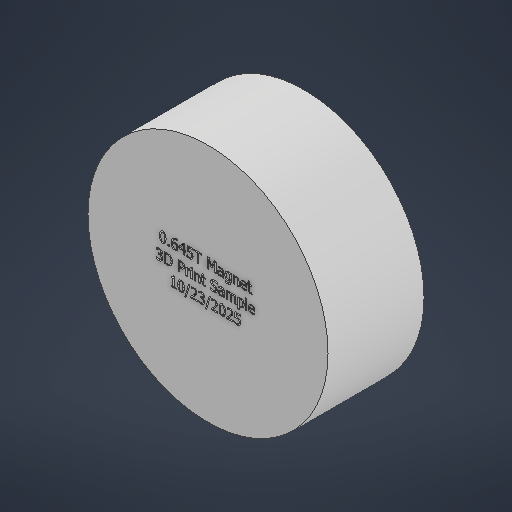
# Autodesk Inventor part: Sample_Magnet
Saved by Autodesk Inventor 2026.1 (Build 301233000, 233)
## iProperties
Created: 2025-10-23
Part Number: Sample_Magnet
Material: Generic
Document SubType Name: Modeling
Designer: usman
Density: 1 g/cm^3
Appearance: Default
Author: usman
Autodesk Inventor part; units mm, degrees
ref_plane "YZ Plane" through (0, 0, 0) normal (1, 0, 0) x (0, 1, 0)
ref_plane "XZ Plane" through (0, 0, 0) normal (0, 1, 0) x (-1, 0, 0)
ref_plane "XY Plane" through (0, 0, 0) normal (0, 0, 1) x (1, 0, 0)
sketch "Sketch1" plane through (0, 0, 0) normal (0, 0, 1) x (1, 0, 0)
  circle A0 centre (0, 0) radius 37.5
  dimension "d0" = 75
  constraints: 1 centre point, 1 coincident
  measures "d0" diameter of A0
extrude "Extrusion1" add sketch "Sketch1" along normal blind 30
sketch "Sketch2" plane through (0, 0, 30) normal (0, 0, 1) x (1, 0, 0)
  line L0 (-22.0603, 24.5034) -> (20.4794, 24.5034) construction
  line L1 (20.4794, 24.5034) -> (20.4794, -24.5034) construction
  line L2 (20.4794, -24.5034) -> (-22.0603, -24.5034) construction
  line L3 (-22.0603, -24.5034) -> (-22.0603, 24.5034) construction
  spline S0 degree 2 poles (-13.0981, 5.5402) (-13.0981, 4.686) (-13.5946, 3.8858) (-14.1118, 3.8858) knots 0 0 0 1 2 2 2
  spline S1 degree 2 poles (-14.1118, 3.8858) (-14.6367, 3.8858) (-15.1281, 4.7014) (-15.1281, 5.5376) knots 0 0 0 1 2 2 2
  spline S2 degree 2 poles (-15.1281, 5.5376) (-15.1281, 6.397) (-14.6315, 7.192) (-14.1118, 7.192) knots 0 0 0 1 2 2 2
  spline S3 degree 2 poles (-14.1118, 7.192) (-13.5895, 7.192) (-13.0981, 6.3686) (-13.0981, 5.5402) knots 0 0 0 1 2 2 2
  spline S4 degree 2 poles (-13.6435, 4.5727) (-13.5818, 4.7297) (-13.5303, 5.2134) (-13.5303, 5.5402) knots 0 0 0 1 2 2 2
  spline S5 degree 2 poles (-13.5303, 5.5402) (-13.5303, 5.8669) (-13.5818, 6.3481) (-13.6461, 6.5102) knots 0 0 0 1 2 2 2
  spline S6 degree 2 poles (-13.6461, 6.5102) (-13.7104, 6.6723) (-13.9343, 6.8395) (-14.1118, 6.8395) knots 0 0 0 1 2 2 2
  spline S7 degree 2 poles (-14.1118, 6.8395) (-14.2893, 6.8395) (-14.5183, 6.6723) (-14.5852, 6.505) knots 0 0 0 1 2 2 2
  spline S8 degree 2 poles (-14.5852, 6.505) (-14.6495, 6.3429) (-14.6959, 5.8489) (-14.6959, 5.5376) knots 0 0 0 1 2 2 2
  spline S9 degree 2 poles (-14.6959, 5.5376) (-14.6959, 5.2031) (-14.6547, 4.7554) (-14.5878, 4.5805) knots 0 0 0 1 2 2 2
  spline S10 degree 2 poles (-14.5878, 4.5805) (-14.526, 4.4158) (-14.297, 4.2383) (-14.1118, 4.2383) knots 0 0 0 1 2 2 2
  spline S11 degree 2 poles (-14.1118, 4.2383) (-13.9368, 4.2383) (-13.7078, 4.4055) (-13.6435, 4.5727) knots 0 0 0 1 2 2 2
  line L4 (-12.0097, 3.9527) -> (-12.5192, 3.9527)
  line L5 (-12.5192, 3.9527) -> (-12.5192, 4.5599)
  line L6 (-12.5192, 4.5599) -> (-12.0097, 4.5599)
  line L7 (-12.0097, 4.5599) -> (-12.0097, 3.9527)
  spline S12 degree 2 poles (-9.3622, 4.9818) (-9.3622, 4.7374) (-9.5243, 4.3232) (-9.6606, 4.1842) knots 0 0 0 1 2 2 2
  spline S13 degree 2 poles (-9.6606, 4.1842) (-9.8021, 4.0376) (-10.1572, 3.8858) (-10.3708, 3.8858) knots 0 0 0 1 2 2 2
  spline S14 degree 2 poles (-10.3708, 3.8858) (-10.5843, 3.8858) (-10.9368, 4.0299) (-11.0706, 4.1739) knots 0 0 0 1 2 2 2
  spline S15 degree 2 poles (-11.0706, 4.1739) (-11.2353, 4.3463) (-11.4205, 4.9252) (-11.4205, 5.3472) knots 0 0 0 1 2 2 2
  spline S16 degree 2 poles (-11.4205, 5.3472) (-11.4205, 5.7614) (-11.2507, 6.4278) (-11.0732, 6.6748) knots 0 0 0 1 2 2 2
  spline S17 degree 2 poles (-11.0732, 6.6748) (-10.9008, 6.9167) (-10.3553, 7.1868) (-9.9977, 7.1868) knots 0 0 0 1 2 2 2
  spline S18 degree 2 poles (-9.9977, 7.1868) (-9.8922, 7.1868) (-9.7069, 7.1663) (-9.6375, 7.1431) knots 0 0 0 1 2 2 2
  line L8 (-9.6375, 7.1431) -> (-9.6375, 6.734)
  line L9 (-9.6375, 6.734) -> (-9.6555, 6.734)
  spline S19 degree 2 poles (-9.6555, 6.734) (-9.7147, 6.7649) (-9.9308, 6.8189) (-10.0543, 6.8189) knots 0 0 0 1 2 2 2
  spline S20 degree 2 poles (-10.0543, 6.8189) (-10.4505, 6.8189) (-10.9368, 6.2837) (-10.9831, 5.7589) knots 0 0 0 1 2 2 2
  spline S21 degree 2 poles (-10.9831, 5.7589) (-10.8313, 5.8644) (-10.5123, 5.9801) (-10.3219, 5.9801) knots 0 0 0 1 2 2 2
  spline S22 degree 2 poles (-10.3219, 5.9801) (-10.1366, 5.9801) (-9.8587, 5.9055) (-9.7069, 5.7923) knots 0 0 0 1 2 2 2
  spline S23 degree 2 poles (-9.7069, 5.7923) (-9.532, 5.6611) (-9.3622, 5.2546) (-9.3622, 4.9818) knots 0 0 0 1 2 2 2
  spline S24 degree 2 poles (-9.7944, 4.9638) (-9.7944, 5.1594) (-9.8973, 5.4244) (-10.0105, 5.517) knots 0 0 0 1 2 2 2
  spline S25 degree 2 poles (-10.0105, 5.517) (-10.0954, 5.5839) (-10.3064, 5.6276) (-10.4171, 5.6276) knots 0 0 0 1 2 2 2
  spline S26 degree 2 poles (-10.4171, 5.6276) (-10.5663, 5.6276) (-10.8467, 5.5376) (-10.9831, 5.4527) knots 0 0 0 1 2 2 2
  spline S27 degree 2 poles (-10.9831, 5.4527) (-10.9857, 5.4064) (-10.9908, 5.3189) (-10.9908, 5.252) knots 0 0 0 1 2 2 2
  spline S28 degree 2 poles (-10.9908, 5.252) (-10.9908, 4.9227) (-10.8622, 4.5187) (-10.7644, 4.4132) knots 0 0 0 1 2 2 2
  spline S29 degree 2 poles (-10.7644, 4.4132) (-10.6744, 4.3129) (-10.4788, 4.2331) (-10.3682, 4.2331) knots 0 0 0 1 2 2 2
  spline S30 degree 2 poles (-10.3682, 4.2331) (-10.1109, 4.2331) (-9.7944, 4.5985) (-9.7944, 4.9638) knots 0 0 0 1 2 2 2
  line L10 (-6.9436, 5.0436) -> (-7.3218, 5.0436)
  line L11 (-7.3218, 5.0436) -> (-7.3218, 3.9527)
  line L12 (-7.3218, 3.9527) -> (-7.7309, 3.9527)
  line L13 (-7.7309, 3.9527) -> (-7.7309, 5.0436)
  line L14 (-7.7309, 5.0436) -> (-9.1332, 5.0436)
  line L15 (-9.1332, 5.0436) -> (-9.1332, 5.4913)
  line L16 (-9.1332, 5.4913) -> (-7.7129, 7.1277)
  line L17 (-7.7129, 7.1277) -> (-7.3218, 7.1277)
  line L18 (-7.3218, 7.1277) -> (-7.3218, 5.3858)
  line L19 (-7.3218, 5.3858) -> (-6.9436, 5.3858)
  line L20 (-6.9436, 5.3858) -> (-6.9436, 5.0436)
  line L21 (-7.7309, 5.3858) -> (-7.7309, 6.6259)
  line L22 (-7.7309, 6.6259) -> (-8.7987, 5.3858)
  line L23 (-8.7987, 5.3858) -> (-7.7309, 5.3858)
  spline S31 degree 2 poles (-4.6794, 4.9613) (-4.6794, 4.7323) (-4.8261, 4.3412) (-4.9599, 4.1971) knots 0 0 0 1 2 2 2
  spline S32 degree 2 poles (-4.9599, 4.1971) (-5.0937, 4.053) (-5.4925, 3.8858) (-5.7395, 3.8858) knots 0 0 0 1 2 2 2
  spline S33 degree 2 poles (-5.7395, 3.8858) (-5.9659, 3.8858) (-6.4084, 3.9861) (-6.5705, 4.0659) knots 0 0 0 1 2 2 2
  line L24 (-6.5705, 4.0659) -> (-6.5705, 4.5161)
  line L25 (-6.5705, 4.5161) -> (-6.5397, 4.5161)
  spline S34 degree 2 poles (-6.5397, 4.5161) (-6.4908, 4.4801) (-6.3081, 4.3875) (-6.1975, 4.3463) knots 0 0 0 1 2 2 2
  spline S35 degree 2 poles (-6.1975, 4.3463) (-6.0714, 4.3026) (-5.863, 4.2537) (-5.7318, 4.2537) knots 0 0 0 1 2 2 2
  spline S36 degree 2 poles (-5.7318, 4.2537) (-5.6031, 4.2537) (-5.3612, 4.3463) (-5.2738, 4.4467) knots 0 0 0 1 2 2 2
  spline S37 degree 2 poles (-5.2738, 4.4467) (-5.194, 4.5419) (-5.1117, 4.794) (-5.1117, 4.9638) knots 0 0 0 1 2 2 2
  spline S38 degree 2 poles (-5.1117, 4.9638) (-5.1117, 5.1336) (-5.2043, 5.3498) (-5.2918, 5.4218) knots 0 0 0 1 2 2 2
  spline S39 degree 2 poles (-5.2918, 5.4218) (-5.3818, 5.5016) (-5.6494, 5.5685) (-5.8115, 5.5685) knots 0 0 0 1 2 2 2
  spline S40 degree 2 poles (-5.8115, 5.5685) (-5.9865, 5.5685) (-6.3338, 5.5144) (-6.4393, 5.4913) knots 0 0 0 1 2 2 2
  line L26 (-6.4393, 5.4913) -> (-6.4393, 7.1277)
  line L27 (-6.4393, 7.1277) -> (-4.6974, 7.1277)
  line L28 (-4.6974, 7.1277) -> (-4.6974, 6.7546)
  line L29 (-4.6974, 6.7546) -> (-6.0302, 6.7546)
  line L30 (-6.0302, 6.7546) -> (-6.0302, 5.9081)
  spline S41 degree 2 poles (-6.0302, 5.9081) (-5.953, 5.9184) (-5.8038, 5.9261) (-5.742, 5.9261) knots 0 0 0 1 2 2 2
  spline S42 degree 2 poles (-5.742, 5.9261) (-5.4976, 5.9261) (-5.1606, 5.8463) (-5.0062, 5.728) knots 0 0 0 1 2 2 2
  spline S43 degree 2 poles (-5.0062, 5.728) (-4.8492, 5.6096) (-4.6794, 5.2494) (-4.6794, 4.9613) knots 0 0 0 1 2 2 2
  line L31 (-3.3904, 3.9527) -> (-3.3904, 6.752)
  line L32 (-3.3904, 6.752) -> (-4.4556, 6.752)
  line L33 (-4.4556, 6.752) -> (-4.4556, 7.1277)
  line L34 (-4.4556, 7.1277) -> (-1.9032, 7.1277)
  line L35 (-1.9032, 7.1277) -> (-1.9032, 6.752)
  line L36 (-1.9032, 6.752) -> (-2.9684, 6.752)
  line L37 (-2.9684, 6.752) -> (-2.9684, 3.9527)
  line L38 (-2.9684, 3.9527) -> (-3.3904, 3.9527)
  line L39 (2.5042, 3.9527) -> (2.0822, 3.9527)
  line L40 (2.0822, 3.9527) -> (2.0822, 6.6877)
  line L41 (2.0822, 6.6877) -> (1.2538, 4.8275)
  line L42 (1.2538, 4.8275) -> (0.9965, 4.8275)
  line L43 (0.9965, 4.8275) -> (0.1757, 6.6877)
  line L44 (0.1757, 6.6877) -> (0.1757, 3.9527)
  line L45 (0.1757, 3.9527) -> (-0.218, 3.9527)
  line L46 (-0.218, 3.9527) -> (-0.218, 7.1277)
  line L47 (-0.218, 7.1277) -> (0.3584, 7.1277)
  line L48 (0.3584, 7.1277) -> (1.1508, 5.3601)
  line L49 (1.1508, 5.3601) -> (1.9176, 7.1277)
  line L50 (1.9176, 7.1277) -> (2.5042, 7.1277)
  line L51 (2.5042, 7.1277) -> (2.5042, 3.9527)
  spline S44 degree 2 poles (4.4442, 4.2048) (4.3953, 4.1688) (4.2306, 4.0401) (4.1535, 4.0016) knots 0 0 0 1 2 2 2
  spline S45 degree 2 poles (4.1535, 4.0016) (4.048, 3.9449) (3.8499, 3.8858) (3.6697, 3.8858) knots 0 0 0 1 2 2 2
  spline S46 degree 2 poles (3.6697, 3.8858) (3.5231, 3.8858) (3.2581, 3.9964) (3.1577, 4.0967) knots 0 0 0 1 2 2 2
  spline S47 degree 2 poles (3.1577, 4.0967) (3.0625, 4.1945) (2.9468, 4.4827) (2.9468, 4.6422) knots 0 0 0 1 2 2 2
  spline S48 degree 2 poles (2.9468, 4.6422) (2.9468, 4.8892) (3.1552, 5.2391) (3.3816, 5.3395) knots 0 0 0 1 2 2 2
  spline S49 degree 2 poles (3.3816, 5.3395) (3.5823, 5.4321) (4.1277, 5.5016) (4.4442, 5.5196) knots 0 0 0 1 2 2 2
  line L52 (4.4442, 5.5196) -> (4.4442, 5.5968)
  spline S50 degree 2 poles (4.4442, 5.5968) (4.4442, 5.7357) (4.3593, 5.9081) (4.2821, 5.957) knots 0 0 0 1 2 2 2
  spline S51 degree 2 poles (4.2821, 5.957) (4.2049, 6.0059) (3.9836, 6.0367) (3.8653, 6.0367) knots 0 0 0 1 2 2 2
  spline S52 degree 2 poles (3.8653, 6.0367) (3.7264, 6.0367) (3.3507, 5.9544) (3.1629, 5.8746) knots 0 0 0 1 2 2 2
  line L53 (3.1629, 5.8746) -> (3.1397, 5.8746)
  line L54 (3.1397, 5.8746) -> (3.1397, 6.2837)
  spline S53 degree 2 poles (3.1397, 6.2837) (3.2504, 6.3146) (3.6646, 6.3918) (3.8679, 6.3918) knots 0 0 0 1 2 2 2
  spline S54 degree 2 poles (3.8679, 6.3918) (4.1149, 6.3918) (4.4519, 6.3146) (4.5857, 6.2143) knots 0 0 0 1 2 2 2
  spline S55 degree 2 poles (4.5857, 6.2143) (4.7169, 6.1165) (4.8456, 5.8052) (4.8456, 5.5813) knots 0 0 0 1 2 2 2
  line L55 (4.8456, 5.5813) -> (4.8456, 3.9527)
  line L56 (4.8456, 3.9527) -> (4.4442, 3.9527)
  line L57 (4.4442, 3.9527) -> (4.4442, 4.2048)
  line L58 (4.4442, 4.5393) -> (4.4442, 5.2005)
  spline S56 degree 2 poles (4.4442, 5.2005) (4.3001, 5.1877) (3.8653, 5.1439) (3.7289, 5.1028) knots 0 0 0 1 2 2 2
  spline S57 degree 2 poles (3.7289, 5.1028) (3.5694, 5.0539) (3.361, 4.8506) (3.361, 4.6705) knots 0 0 0 1 2 2 2
  spline S58 degree 2 poles (3.361, 4.6705) (3.361, 4.4647) (3.5926, 4.2563) (3.8138, 4.2563) knots 0 0 0 1 2 2 2
  spline S59 degree 2 poles (3.8138, 4.2563) (4.0017, 4.2563) (4.3104, 4.4184) (4.4442, 4.5393) knots 0 0 0 1 2 2 2
  spline S60 degree 2 poles (5.494, 3.5719) (5.5351, 3.5539) (5.6921, 3.4973) (5.7924, 3.4741) knots 0 0 0 1 2 2 2
  spline S61 degree 2 poles (5.7924, 3.4741) (5.9031, 3.4458) (6.0909, 3.4123) (6.2015, 3.4123) knots 0 0 0 1 2 2 2
  spline S62 degree 2 poles (6.2015, 3.4123) (6.3868, 3.4123) (6.6441, 3.5101) (6.7161, 3.5976) knots 0 0 0 1 2 2 2
  spline S63 degree 2 poles (6.7161, 3.5976) (6.7856, 3.6851) (6.8396, 3.9141) (6.8396, 4.0607) knots 0 0 0 1 2 2 2
  line L59 (6.8396, 4.0607) -> (6.8396, 4.2691)
  spline S64 degree 2 poles (6.8396, 4.2691) (6.6775, 4.1276) (6.3662, 3.9938) (6.132, 3.9938) knots 0 0 0 1 2 2 2
  spline S65 degree 2 poles (6.132, 3.9938) (5.7255, 3.9938) (5.2444, 4.5985) (5.2444, 5.1671) knots 0 0 0 1 2 2 2
  spline S66 degree 2 poles (5.2444, 5.1671) (5.2444, 5.463) (5.4116, 5.921) (5.5506, 6.0831) knots 0 0 0 1 2 2 2
  spline S67 degree 2 poles (5.5506, 6.0831) (5.6844, 6.2349) (6.0523, 6.4021) (6.2478, 6.4021) knots 0 0 0 1 2 2 2
  spline S68 degree 2 poles (6.2478, 6.4021) (6.4331, 6.4021) (6.7032, 6.3146) (6.8396, 6.2349) knots 0 0 0 1 2 2 2
  line L60 (6.8396, 6.2349) -> (6.8628, 6.3352)
  line L61 (6.8628, 6.3352) -> (7.241, 6.3352)
  line L62 (7.241, 6.3352) -> (7.241, 4.2254)
  spline S69 degree 2 poles (7.241, 4.2254) (7.241, 3.6182) (6.7135, 3.0521) (6.1706, 3.0521) knots 0 0 0 1 2 2 2
  spline S70 degree 2 poles (6.1706, 3.0521) (5.9957, 3.0521) (5.6303, 3.1087) (5.4734, 3.1551) knots 0 0 0 1 2 2 2
  line L63 (5.4734, 3.1551) -> (5.4734, 3.5719)
  line L64 (5.4734, 3.5719) -> (5.494, 3.5719)
  line L65 (6.8396, 4.5985) -> (6.8396, 5.9081)
  spline S71 degree 2 poles (6.8396, 5.9081) (6.6904, 5.9801) (6.4382, 6.0419) (6.3122, 6.0419) knots 0 0 0 1 2 2 2
  spline S72 degree 2 poles (6.3122, 6.0419) (6.0085, 6.0419) (5.6586, 5.5942) (5.6586, 5.1748) knots 0 0 0 1 2 2 2
  spline S73 degree 2 poles (5.6586, 5.1748) (5.6586, 4.7786) (5.9236, 4.3643) (6.2221, 4.3643) knots 0 0 0 1 2 2 2
  spline S74 degree 2 poles (6.2221, 4.3643) (6.379, 4.3643) (6.7084, 4.4878) (6.8396, 4.5985) knots 0 0 0 1 2 2 2
  line L66 (9.693, 3.9527) -> (9.2916, 3.9527)
  line L67 (9.2916, 3.9527) -> (9.2916, 5.3112)
  spline S75 degree 2 poles (9.2916, 5.3112) (9.2916, 5.4758) (9.2607, 5.7589) (9.2144, 5.8438) knots 0 0 0 1 2 2 2
  spline S76 degree 2 poles (9.2144, 5.8438) (9.1655, 5.9338) (8.9906, 6.0213) (8.8413, 6.0213) knots 0 0 0 1 2 2 2
  spline S77 degree 2 poles (8.8413, 6.0213) (8.6921, 6.0213) (8.3756, 5.8618) (8.2238, 5.7331) knots 0 0 0 1 2 2 2
  line L68 (8.2238, 5.7331) -> (8.2238, 3.9527)
  line L69 (8.2238, 3.9527) -> (7.8225, 3.9527)
  line L70 (7.8225, 3.9527) -> (7.8225, 6.3352)
  line L71 (7.8225, 6.3352) -> (8.2238, 6.3352)
  line L72 (8.2238, 6.3352) -> (8.2238, 6.0702)
  spline S78 degree 2 poles (8.2238, 6.0702) (8.4039, 6.2323) (8.7513, 6.4021) (8.9468, 6.4021) knots 0 0 0 1 2 2 2
  spline S79 degree 2 poles (8.9468, 6.4021) (9.2968, 6.4021) (9.693, 5.939) (9.693, 5.499) knots 0 0 0 1 2 2 2
  line L73 (9.693, 5.499) -> (9.693, 3.9527)
  spline S80 degree 2 poles (11.2908, 3.8986) (10.7196, 3.8986) (10.0918, 4.5393) (10.0918, 5.1311) knots 0 0 0 1 2 2 2
  spline S81 degree 2 poles (10.0918, 5.1311) (10.0918, 5.7126) (10.7016, 6.4021) (11.193, 6.4021) knots 0 0 0 1 2 2 2
  spline S82 degree 2 poles (11.193, 6.4021) (11.4143, 6.4021) (11.7565, 6.2735) (11.8826, 6.1371) knots 0 0 0 1 2 2 2
  spline S83 degree 2 poles (11.8826, 6.1371) (12.0112, 6.0007) (12.1476, 5.6071) (12.1476, 5.3215) knots 0 0 0 1 2 2 2
  line L74 (12.1476, 5.3215) -> (12.1476, 5.1028)
  line L75 (12.1476, 5.1028) -> (10.4983, 5.1028)
  spline S84 degree 2 poles (10.4983, 5.1028) (10.4983, 4.6885) (10.9151, 4.2486) (11.2856, 4.2486) knots 0 0 0 1 2 2 2
  spline S85 degree 2 poles (11.2856, 4.2486) (11.4169, 4.2486) (11.6716, 4.3077) (11.7745, 4.354) knots 0 0 0 1 2 2 2
  spline S86 degree 2 poles (11.7745, 4.354) (11.8826, 4.4055) (12.0318, 4.4956) (12.0807, 4.5367) knots 0 0 0 1 2 2 2
  line L76 (12.0807, 4.5367) -> (12.1038, 4.5367)
  line L77 (12.1038, 4.5367) -> (12.1038, 4.0993)
  spline S87 degree 2 poles (12.1038, 4.0993) (12.0344, 4.071) (11.8234, 3.9887) (11.741, 3.9655) knots 0 0 0 1 2 2 2
  spline S88 degree 2 poles (11.741, 3.9655) (11.6253, 3.9321) (11.4349, 3.8986) (11.2908, 3.8986) knots 0 0 0 1 2 2 2
  spline S89 degree 2 poles (11.7565, 5.4089) (11.7513, 5.571) (11.6844, 5.8078) (11.6201, 5.8875) knots 0 0 0 1 2 2 2
  spline S90 degree 2 poles (11.6201, 5.8875) (11.5506, 5.9776) (11.3319, 6.0728) (11.1698, 6.0728) knots 0 0 0 1 2 2 2
  spline S91 degree 2 poles (11.1698, 6.0728) (11.0103, 6.0728) (10.7865, 5.9776) (10.6939, 5.8849) knots 0 0 0 1 2 2 2
  spline S92 degree 2 poles (10.6939, 5.8849) (10.6038, 5.7897) (10.5112, 5.5607) (10.4983, 5.4089) knots 0 0 0 1 2 2 2
  line L78 (10.4983, 5.4089) -> (11.7565, 5.4089)
  spline S93 degree 2 poles (13.2745, 3.9064) (12.9477, 3.9064) (12.5798, 4.2794) (12.5798, 4.6834) knots 0 0 0 1 2 2 2
  line L79 (12.5798, 4.6834) -> (12.5798, 6.0033)
  line L80 (12.5798, 6.0033) -> (12.3097, 6.0033)
  line L81 (12.3097, 6.0033) -> (12.3097, 6.3352)
  line L82 (12.3097, 6.3352) -> (12.5798, 6.3352)
  line L83 (12.5798, 6.3352) -> (12.5798, 7.0196)
  line L84 (12.5798, 7.0196) -> (12.9812, 7.0196)
  line L85 (12.9812, 7.0196) -> (12.9812, 6.3352)
  line L86 (12.9812, 6.3352) -> (13.7196, 6.3352)
  line L87 (13.7196, 6.3352) -> (13.7196, 6.0033)
  line L88 (13.7196, 6.0033) -> (12.9812, 6.0033)
  line L89 (12.9812, 6.0033) -> (12.9812, 4.8686)
  spline S94 degree 2 poles (12.9812, 4.8686) (12.9812, 4.6885) (12.9941, 4.4904) (13.0378, 4.4055) knots 0 0 0 1 2 2 2
  spline S95 degree 2 poles (13.0378, 4.4055) (13.0738, 4.3309) (13.2359, 4.2563) (13.3749, 4.2563) knots 0 0 0 1 2 2 2
  spline S96 degree 2 poles (13.3749, 4.2563) (13.4726, 4.2563) (13.6553, 4.3154) (13.6965, 4.3335) knots 0 0 0 1 2 2 2
  line L90 (13.6965, 4.3335) -> (13.7196, 4.3335)
  line L91 (13.7196, 4.3335) -> (13.7196, 3.9732)
  spline S97 degree 2 poles (13.7196, 3.9732) (13.6064, 3.9424) (13.3749, 3.9064) (13.2745, 3.9064) knots 0 0 0 1 2 2 2
  spline S98 degree 2 poles (-15.2259, 1.5991) (-15.3417, 1.5991) (-15.5706, 1.5425) (-15.6813, 1.4987) knots 0 0 0 1 2 2 2
  spline S99 degree 2 poles (-15.6813, 1.4987) (-15.7842, 1.455) (-15.936, 1.3624) (-15.9952, 1.3212) knots 0 0 0 1 2 2 2
  line L92 (-15.9952, 1.3212) -> (-16.0209, 1.3212)
  line L93 (-16.0209, 1.3212) -> (-16.0209, 1.7715)
  spline S100 degree 2 poles (-16.0209, 1.7715) (-15.882, 1.8461) (-15.406, 1.967) (-15.1924, 1.967) knots 0 0 0 1 2 2 2
  spline S101 degree 2 poles (-15.1924, 1.967) (-14.9763, 1.967) (-14.6547, 1.8795) (-14.5235, 1.7869) knots 0 0 0 1 2 2 2
  spline S102 degree 2 poles (-14.5235, 1.7869) (-14.3845, 1.6866) (-14.2404, 1.3958) (-14.2404, 1.2003) knots 0 0 0 1 2 2 2
  spline S103 degree 2 poles (-14.2404, 1.2003) (-14.2404, 0.9378) (-14.5852, 0.5416) (-14.8271, 0.4901) knots 0 0 0 1 2 2 2
  line L94 (-14.8271, 0.4901) -> (-14.8271, 0.4593)
  spline S104 degree 2 poles (-14.8271, 0.4593) (-14.7267, 0.4387) (-14.4977, 0.3461) (-14.4, 0.2534) knots 0 0 0 1 2 2 2
  spline S105 degree 2 poles (-14.4, 0.2534) (-14.3022, 0.1634) (-14.1787, -0.1248) (-14.1787, -0.3332) knots 0 0 0 1 2 2 2
  spline S106 degree 2 poles (-14.1787, -0.3332) (-14.1787, -0.5467) (-14.3253, -0.9095) (-14.4591, -1.0485) knots 0 0 0 1 2 2 2
  spline S107 degree 2 poles (-14.4591, -1.0485) (-14.5981, -1.1926) (-14.9917, -1.3418) (-15.2413, -1.3418) knots 0 0 0 1 2 2 2
  spline S108 degree 2 poles (-15.2413, -1.3418) (-15.4806, -1.3418) (-15.9489, -1.226) (-16.1084, -1.1462) knots 0 0 0 1 2 2 2
  line L95 (-16.1084, -1.1462) -> (-16.1084, -0.696)
  line L96 (-16.1084, -0.696) -> (-16.0775, -0.696)
  spline S109 degree 2 poles (-16.0775, -0.696) (-15.9437, -0.7937) (-15.4909, -0.9739) (-15.267, -0.9739) knots 0 0 0 1 2 2 2
  spline S110 degree 2 poles (-15.267, -0.9739) (-15.1358, -0.9739) (-14.8734, -0.8915) (-14.7859, -0.7963) knots 0 0 0 1 2 2 2
  spline S111 degree 2 poles (-14.7859, -0.7963) (-14.701, -0.7011) (-14.6109, -0.4747) (-14.6109, -0.3023) knots 0 0 0 1 2 2 2
  spline S112 degree 2 poles (-14.6109, -0.3023) (-14.6109, -0.1299) (-14.7113, 0.0939) (-14.8013, 0.1582) knots 0 0 0 1 2 2 2
  spline S113 degree 2 poles (-14.8013, 0.1582) (-14.8914, 0.2226) (-15.1358, 0.2714) (-15.2799, 0.2714) knots 0 0 0 1 2 2 2
  line L97 (-15.2799, 0.2714) -> (-15.46, 0.2714)
  line L98 (-15.46, 0.2714) -> (-15.46, 0.6239)
  line L99 (-15.46, 0.6239) -> (-15.3185, 0.6239)
  spline S114 degree 2 poles (-15.3185, 0.6239) (-15.0329, 0.6239) (-14.6727, 0.8967) (-14.6727, 1.1565) knots 0 0 0 1 2 2 2
  spline S115 degree 2 poles (-14.6727, 1.1565) (-14.6727, 1.2775) (-14.7653, 1.4498) (-14.8399, 1.5013) knots 0 0 0 1 2 2 2
  spline S116 degree 2 poles (-14.8399, 1.5013) (-14.9197, 1.5553) (-15.1152, 1.5991) (-15.2259, 1.5991) knots 0 0 0 1 2 2 2
  spline S117 degree 2 poles (-11.1066, 0.31) (-11.1066, -0.1248) (-11.4591, -0.8246) (-11.755, -1.0202) knots 0 0 0 1 2 2 2
  spline S118 degree 2 poles (-11.755, -1.0202) (-11.9968, -1.172) (-12.4934, -1.2749) (-12.8794, -1.2749) knots 0 0 0 1 2 2 2
  line L100 (-12.8794, -1.2749) -> (-13.6101, -1.2749)
  line L101 (-13.6101, -1.2749) -> (-13.6101, 1.9001)
  line L102 (-13.6101, 1.9001) -> (-12.8871, 1.9001)
  spline S119 degree 2 poles (-12.8871, 1.9001) (-12.4394, 1.9001) (-11.9299, 1.7663) (-11.7498, 1.648) knots 0 0 0 1 2 2 2
  spline S120 degree 2 poles (-11.7498, 1.648) (-11.4437, 1.4447) (-11.1066, 0.7732) (-11.1066, 0.31) knots 0 0 0 1 2 2 2
  spline S121 degree 2 poles (-11.5466, 0.3152) (-11.5466, 0.6805) (-11.7884, 1.1977) (-12.0277, 1.3444) knots 0 0 0 1 2 2 2
  spline S122 degree 2 poles (-12.0277, 1.3444) (-12.1975, 1.4447) (-12.5809, 1.5348) (-12.8665, 1.5348) knots 0 0 0 1 2 2 2
  line L103 (-12.8665, 1.5348) -> (-13.1881, 1.5348)
  line L104 (-13.1881, 1.5348) -> (-13.1881, -0.9095)
  line L105 (-13.1881, -0.9095) -> (-12.8665, -0.9095)
  spline S123 degree 2 poles (-12.8665, -0.9095) (-12.586, -0.9095) (-12.1615, -0.8195) (-11.9891, -0.6986) knots 0 0 0 1 2 2 2
  spline S124 degree 2 poles (-11.9891, -0.6986) (-11.7679, -0.5493) (-11.5466, -0.0553) (-11.5466, 0.3152) knots 0 0 0 1 2 2 2
  spline S125 degree 2 poles (-7.2781, 0.943) (-7.2781, 0.7371) (-7.4247, 0.3666) (-7.556, 0.238) knots 0 0 0 1 2 2 2
  spline S126 degree 2 poles (-7.556, 0.238) (-7.7206, 0.0759) (-8.1657, -0.0913) (-8.5054, -0.0913) knots 0 0 0 1 2 2 2
  line L106 (-8.5054, -0.0913) -> (-8.863, -0.0913)
  line L107 (-8.863, -0.0913) -> (-8.863, -1.2749)
  line L108 (-8.863, -1.2749) -> (-9.285, -1.2749)
  line L109 (-9.285, -1.2749) -> (-9.285, 1.9001)
  line L110 (-9.285, 1.9001) -> (-8.4874, 1.9001)
  spline S127 degree 2 poles (-8.4874, 1.9001) (-8.2043, 1.9001) (-7.8081, 1.8075) (-7.6563, 1.702) knots 0 0 0 1 2 2 2
  spline S128 degree 2 poles (-7.6563, 1.702) (-7.4788, 1.5811) (-7.2781, 1.208) (-7.2781, 0.943) knots 0 0 0 1 2 2 2
  spline S129 degree 2 poles (-7.7181, 0.9301) (-7.7181, 1.0948) (-7.8313, 1.3366) (-7.947, 1.4138) knots 0 0 0 1 2 2 2
  spline S130 degree 2 poles (-7.947, 1.4138) (-8.0474, 1.4807) (-8.315, 1.5348) (-8.5131, 1.5348) knots 0 0 0 1 2 2 2
  line L111 (-8.5131, 1.5348) -> (-8.863, 1.5348)
  line L112 (-8.863, 1.5348) -> (-8.863, 0.2689)
  line L113 (-8.863, 0.2689) -> (-8.5748, 0.2689)
  spline S131 degree 2 poles (-8.5748, 0.2689) (-8.3175, 0.2689) (-8.0011, 0.3512) (-7.8982, 0.4593) knots 0 0 0 1 2 2 2
  spline S132 degree 2 poles (-7.8982, 0.4593) (-7.803, 0.5545) (-7.7181, 0.7783) (-7.7181, 0.9301) knots 0 0 0 1 2 2 2
  line L114 (-5.6443, 0.678) -> (-5.6649, 0.678)
  spline S133 degree 2 poles (-5.6649, 0.678) (-5.7112, 0.6908) (-5.8115, 0.696) (-5.881, 0.696) knots 0 0 0 1 2 2 2
  spline S134 degree 2 poles (-5.881, 0.696) (-6.0431, 0.696) (-6.3621, 0.5545) (-6.5062, 0.4155) knots 0 0 0 1 2 2 2
  line L115 (-6.5062, 0.4155) -> (-6.5062, -1.2749)
  line L116 (-6.5062, -1.2749) -> (-6.9076, -1.2749)
  line L117 (-6.9076, -1.2749) -> (-6.9076, 1.1076)
  line L118 (-6.9076, 1.1076) -> (-6.5062, 1.1076)
  line L119 (-6.5062, 1.1076) -> (-6.5062, 0.7526)
  spline S135 degree 2 poles (-6.5062, 0.7526) (-6.2875, 0.9481) (-5.9607, 1.1076) (-5.8064, 1.1076) knots 0 0 0 1 2 2 2
  spline S136 degree 2 poles (-5.8064, 1.1076) (-5.7446, 1.1076) (-5.6829, 1.1025) (-5.6443, 1.0948) knots 0 0 0 1 2 2 2
  line L120 (-5.6443, 1.0948) -> (-5.6443, 0.678)
  line L121 (-4.9238, -1.2749) -> (-5.3252, -1.2749)
  line L122 (-5.3252, -1.2749) -> (-5.3252, 1.1076)
  line L123 (-5.3252, 1.1076) -> (-4.9238, 1.1076)
  line L124 (-4.9238, 1.1076) -> (-4.9238, -1.2749)
  line L125 (-4.8955, 1.5039) -> (-5.351, 1.5039)
  line L126 (-5.351, 1.5039) -> (-5.351, 1.9207)
  line L127 (-5.351, 1.9207) -> (-4.8955, 1.9207)
  line L128 (-4.8955, 1.9207) -> (-4.8955, 1.5039)
  line L129 (-2.4641, -1.2749) -> (-2.8655, -1.2749)
  line L130 (-2.8655, -1.2749) -> (-2.8655, 0.0836)
  spline S137 degree 2 poles (-2.8655, 0.0836) (-2.8655, 0.2483) (-2.8964, 0.5313) (-2.9427, 0.6162) knots 0 0 0 1 2 2 2
  spline S138 degree 2 poles (-2.9427, 0.6162) (-2.9916, 0.7063) (-3.1665, 0.7938) (-3.3158, 0.7938) knots 0 0 0 1 2 2 2
  spline S139 degree 2 poles (-3.3158, 0.7938) (-3.465, 0.7938) (-3.7815, 0.6342) (-3.9333, 0.5056) knots 0 0 0 1 2 2 2
  line L131 (-3.9333, 0.5056) -> (-3.9333, -1.2749)
  line L132 (-3.9333, -1.2749) -> (-4.3346, -1.2749)
  line L133 (-4.3346, -1.2749) -> (-4.3346, 1.1076)
  line L134 (-4.3346, 1.1076) -> (-3.9333, 1.1076)
  line L135 (-3.9333, 1.1076) -> (-3.9333, 0.8426)
  spline S140 degree 2 poles (-3.9333, 0.8426) (-3.7532, 1.0047) (-3.4058, 1.1745) (-3.2103, 1.1745) knots 0 0 0 1 2 2 2
  spline S141 degree 2 poles (-3.2103, 1.1745) (-2.8604, 1.1745) (-2.4641, 0.7114) (-2.4641, 0.2714) knots 0 0 0 1 2 2 2
  line L136 (-2.4641, 0.2714) -> (-2.4641, -1.2749)
  spline S142 degree 2 poles (-1.1802, -1.3212) (-1.507, -1.3212) (-1.8749, -0.9481) (-1.8749, -0.5442) knots 0 0 0 1 2 2 2
  line L137 (-1.8749, -0.5442) -> (-1.8749, 0.7757)
  line L138 (-1.8749, 0.7757) -> (-2.1451, 0.7757)
  line L139 (-2.1451, 0.7757) -> (-2.1451, 1.1076)
  line L140 (-2.1451, 1.1076) -> (-1.8749, 1.1076)
  line L141 (-1.8749, 1.1076) -> (-1.8749, 1.792)
  line L142 (-1.8749, 1.792) -> (-1.4735, 1.792)
  line L143 (-1.4735, 1.792) -> (-1.4735, 1.1076)
  line L144 (-1.4735, 1.1076) -> (-0.7351, 1.1076)
  line L145 (-0.7351, 1.1076) -> (-0.7351, 0.7757)
  line L146 (-0.7351, 0.7757) -> (-1.4735, 0.7757)
  line L147 (-1.4735, 0.7757) -> (-1.4735, -0.3589)
  spline S143 degree 2 poles (-1.4735, -0.3589) (-1.4735, -0.539) (-1.4607, -0.7371) (-1.4169, -0.8221) knots 0 0 0 1 2 2 2
  spline S144 degree 2 poles (-1.4169, -0.8221) (-1.3809, -0.8967) (-1.2188, -0.9713) (-1.0799, -0.9713) knots 0 0 0 1 2 2 2
  spline S145 degree 2 poles (-1.0799, -0.9713) (-0.9821, -0.9713) (-0.7994, -0.9121) (-0.7583, -0.8941) knots 0 0 0 1 2 2 2
  line L148 (-0.7583, -0.8941) -> (-0.7351, -0.8941)
  line L149 (-0.7351, -0.8941) -> (-0.7351, -1.2543)
  spline S146 degree 2 poles (-0.7351, -1.2543) (-0.8483, -1.2852) (-1.0799, -1.3212) (-1.1802, -1.3212) knots 0 0 0 1 2 2 2
  spline S147 degree 2 poles (1.8404, -1.3315) (1.4956, -1.3315) (1.0119, -1.1874) (0.7984, -1.0845) knots 0 0 0 1 2 2 2
  line L150 (0.7984, -1.0845) -> (0.7984, -0.5545)
  line L151 (0.7984, -0.5545) -> (0.8292, -0.5545)
  spline S148 degree 2 poles (0.8292, -0.5545) (1.0376, -0.75) (1.5651, -0.9661) (1.8095, -0.9661) knots 0 0 0 1 2 2 2
  spline S149 degree 2 poles (1.8095, -0.9661) (2.1594, -0.9661) (2.5171, -0.6754) (2.5171, -0.4361) knots 0 0 0 1 2 2 2
  spline S150 degree 2 poles (2.5171, -0.4361) (2.5171, -0.2457) (2.3292, -0.009) (2.126, 0.0502) knots 0 0 0 1 2 2 2
  spline S151 degree 2 poles (2.126, 0.0502) (1.9793, 0.0913) (1.7349, 0.1479) (1.5522, 0.1943) knots 0 0 0 1 2 2 2
  spline S152 degree 2 poles (1.5522, 0.1943) (1.3876, 0.238) (1.1277, 0.3692) (1.0273, 0.4747) knots 0 0 0 1 2 2 2
  spline S153 degree 2 poles (1.0273, 0.4747) (0.9296, 0.5802) (0.8215, 0.8632) (0.8215, 1.0485) knots 0 0 0 1 2 2 2
  spline S154 degree 2 poles (0.8215, 1.0485) (0.8215, 1.4344) (1.4236, 1.9567) (1.8893, 1.9567) knots 0 0 0 1 2 2 2
  spline S155 degree 2 poles (1.8893, 1.9567) (2.1569, 1.9567) (2.6303, 1.8512) (2.8335, 1.7509) knots 0 0 0 1 2 2 2
  line L152 (2.8335, 1.7509) -> (2.8335, 1.2466)
  line L153 (2.8335, 1.2466) -> (2.8027, 1.2466)
  spline S156 degree 2 poles (2.8027, 1.2466) (2.6509, 1.3855) (2.1774, 1.5914) (1.9176, 1.5914) knots 0 0 0 1 2 2 2
  spline S157 degree 2 poles (1.9176, 1.5914) (1.6243, 1.5914) (1.2615, 1.3161) (1.2615, 1.0922) knots 0 0 0 1 2 2 2
  spline S158 degree 2 poles (1.2615, 1.0922) (1.2615, 0.8915) (1.475, 0.6522) (1.6757, 0.5982) knots 0 0 0 1 2 2 2
  spline S159 degree 2 poles (1.6757, 0.5982) (1.8095, 0.5622) (2.198, 0.4696) (2.3267, 0.431) knots 0 0 0 1 2 2 2
  spline S160 degree 2 poles (2.3267, 0.431) (2.6534, 0.3306) (2.957, -0.0733) (2.957, -0.3692) knots 0 0 0 1 2 2 2
  spline S161 degree 2 poles (2.957, -0.3692) (2.957, -0.557) (2.8052, -0.9173) (2.6689, -1.0433) knots 0 0 0 1 2 2 2
  spline S162 degree 2 poles (2.6689, -1.0433) (2.5171, -1.1823) (2.1311, -1.3315) (1.8404, -1.3315) knots 0 0 0 1 2 2 2
  spline S163 degree 2 poles (4.6835, -1.0227) (4.6346, -1.0588) (4.4699, -1.1874) (4.3927, -1.226) knots 0 0 0 1 2 2 2
  spline S164 degree 2 poles (4.3927, -1.226) (4.2873, -1.2826) (4.0891, -1.3418) (3.909, -1.3418) knots 0 0 0 1 2 2 2
  spline S165 degree 2 poles (3.909, -1.3418) (3.7624, -1.3418) (3.4974, -1.2311) (3.397, -1.1308) knots 0 0 0 1 2 2 2
  spline S166 degree 2 poles (3.397, -1.1308) (3.3018, -1.033) (3.186, -0.7449) (3.186, -0.5853) knots 0 0 0 1 2 2 2
  spline S167 degree 2 poles (3.186, -0.5853) (3.186, -0.3383) (3.3944, 0.0116) (3.6209, 0.1119) knots 0 0 0 1 2 2 2
  spline S168 degree 2 poles (3.6209, 0.1119) (3.8216, 0.2045) (4.367, 0.274) (4.6835, 0.292) knots 0 0 0 1 2 2 2
  line L154 (4.6835, 0.292) -> (4.6835, 0.3692)
  spline S169 degree 2 poles (4.6835, 0.3692) (4.6835, 0.5082) (4.5986, 0.6805) (4.5214, 0.7294) knots 0 0 0 1 2 2 2
  spline S170 degree 2 poles (4.5214, 0.7294) (4.4442, 0.7783) (4.2229, 0.8092) (4.1046, 0.8092) knots 0 0 0 1 2 2 2
  spline S171 degree 2 poles (4.1046, 0.8092) (3.9656, 0.8092) (3.59, 0.7269) (3.4022, 0.6471) knots 0 0 0 1 2 2 2
  line L155 (3.4022, 0.6471) -> (3.379, 0.6471)
  line L156 (3.379, 0.6471) -> (3.379, 1.0562)
  spline S172 degree 2 poles (3.379, 1.0562) (3.4896, 1.0871) (3.9039, 1.1643) (4.1071, 1.1643) knots 0 0 0 1 2 2 2
  spline S173 degree 2 poles (4.1071, 1.1643) (4.3541, 1.1643) (4.6912, 1.0871) (4.825, 0.9867) knots 0 0 0 1 2 2 2
  spline S174 degree 2 poles (4.825, 0.9867) (4.9562, 0.8889) (5.0849, 0.5776) (5.0849, 0.3538) knots 0 0 0 1 2 2 2
  line L157 (5.0849, 0.3538) -> (5.0849, -1.2749)
  line L158 (5.0849, -1.2749) -> (4.6835, -1.2749)
  line L159 (4.6835, -1.2749) -> (4.6835, -1.0227)
  line L160 (4.6835, -0.6883) -> (4.6835, -0.027)
  spline S175 degree 2 poles (4.6835, -0.027) (4.5394, -0.0399) (4.1046, -0.0836) (3.9682, -0.1248) knots 0 0 0 1 2 2 2
  spline S176 degree 2 poles (3.9682, -0.1248) (3.8087, -0.1737) (3.6003, -0.3769) (3.6003, -0.557) knots 0 0 0 1 2 2 2
  spline S177 degree 2 poles (3.6003, -0.557) (3.6003, -0.7629) (3.8318, -0.9713) (4.0531, -0.9713) knots 0 0 0 1 2 2 2
  spline S178 degree 2 poles (4.0531, -0.9713) (4.2409, -0.9713) (4.5497, -0.8092) (4.6835, -0.6883) knots 0 0 0 1 2 2 2
  line L161 (8.3499, -1.2749) -> (8.3499, 0.1042)
  spline S179 degree 2 poles (8.3499, 0.1042) (8.3499, 0.2689) (8.3242, 0.5493) (8.283, 0.6265) knots 0 0 0 1 2 2 2
  spline S180 degree 2 poles (8.283, 0.6265) (8.2419, 0.7114) (8.0849, 0.7938) (7.9485, 0.7938) knots 0 0 0 1 2 2 2
  spline S181 degree 2 poles (7.9485, 0.7938) (7.825, 0.7938) (7.542, 0.6419) (7.3928, 0.4979) knots 0 0 0 1 2 2 2
  spline S182 degree 2 poles (7.3928, 0.4979) (7.3954, 0.4618) (7.4005, 0.3615) (7.4005, 0.2946) knots 0 0 0 1 2 2 2
  line L162 (7.4005, 0.2946) -> (7.4005, -1.2749)
  line L163 (7.4005, -1.2749) -> (6.9991, -1.2749)
  line L164 (6.9991, -1.2749) -> (6.9991, 0.1042)
  spline S183 degree 2 poles (6.9991, 0.1042) (6.9991, 0.2689) (6.9734, 0.5493) (6.9322, 0.6265) knots 0 0 0 1 2 2 2
  spline S184 degree 2 poles (6.9322, 0.6265) (6.8911, 0.7114) (6.7341, 0.7938) (6.5977, 0.7938) knots 0 0 0 1 2 2 2
  spline S185 degree 2 poles (6.5977, 0.7938) (6.4691, 0.7938) (6.1835, 0.6317) (6.0497, 0.5056) knots 0 0 0 1 2 2 2
  line L165 (6.0497, 0.5056) -> (6.0497, -1.2749)
  line L166 (6.0497, -1.2749) -> (5.6483, -1.2749)
  line L167 (5.6483, -1.2749) -> (5.6483, 1.1076)
  line L168 (5.6483, 1.1076) -> (6.0497, 1.1076)
  line L169 (6.0497, 1.1076) -> (6.0497, 0.8452)
  spline S186 degree 2 poles (6.0497, 0.8452) (6.2067, 1.0022) (6.5154, 1.1745) (6.7007, 1.1745) knots 0 0 0 1 2 2 2
  spline S187 degree 2 poles (6.7007, 1.1745) (6.9116, 1.1745) (7.2384, 0.9816) (7.3233, 0.7629) knots 0 0 0 1 2 2 2
  spline S188 degree 2 poles (7.3233, 0.7629) (7.506, 0.9661) (7.8508, 1.1745) (8.0515, 1.1745) knots 0 0 0 1 2 2 2
  spline S189 degree 2 poles (8.0515, 1.1745) (8.2058, 1.1745) (8.458, 1.0793) (8.5506, 0.9713) knots 0 0 0 1 2 2 2
  spline S190 degree 2 poles (8.5506, 0.9713) (8.6458, 0.8632) (8.7513, 0.539) (8.7513, 0.2946) knots 0 0 0 1 2 2 2
  line L170 (8.7513, 0.2946) -> (8.7513, -1.2749)
  line L171 (8.7513, -1.2749) -> (8.3499, -1.2749)
  spline S191 degree 2 poles (11.3114, -0.0193) (11.3114, -0.6162) (10.7427, -1.3212) (10.3079, -1.3212) knots 0 0 0 1 2 2 2
  spline S192 degree 2 poles (10.3079, -1.3212) (10.1304, -1.3212) (9.8577, -1.2389) (9.7161, -1.154) knots 0 0 0 1 2 2 2
  line L172 (9.7161, -1.154) -> (9.7161, -2.1523)
  line L173 (9.7161, -2.1523) -> (9.3148, -2.1523)
  line L174 (9.3148, -2.1523) -> (9.3148, 1.1076)
  line L175 (9.3148, 1.1076) -> (9.7161, 1.1076)
  line L176 (9.7161, 1.1076) -> (9.7161, 0.8581)
  spline S193 degree 2 poles (9.7161, 0.8581) (9.8654, 0.9944) (10.2307, 1.1745) (10.4443, 1.1745) knots 0 0 0 1 2 2 2
  spline S194 degree 2 poles (10.4443, 1.1745) (10.8534, 1.1745) (11.3114, 0.5262) (11.3114, -0.0193) knots 0 0 0 1 2 2 2
  spline S195 degree 2 poles (10.8971, -0.0656) (10.8971, 0.3435) (10.6373, 0.7938) (10.3465, 0.7938) knots 0 0 0 1 2 2 2
  spline S196 degree 2 poles (10.3465, 0.7938) (10.1767, 0.7938) (9.8577, 0.6419) (9.7161, 0.5236) knots 0 0 0 1 2 2 2
  line L177 (9.7161, 0.5236) -> (9.7161, -0.8298)
  spline S197 degree 2 poles (9.7161, -0.8298) (9.8731, -0.9044) (10.0969, -0.961) (10.241, -0.961) knots 0 0 0 1 2 2 2
  spline S198 degree 2 poles (10.241, -0.961) (10.5523, -0.961) (10.8971, -0.503) (10.8971, -0.0656) knots 0 0 0 1 2 2 2
  line L178 (12.1373, -1.2749) -> (11.7359, -1.2749)
  line L179 (11.7359, -1.2749) -> (11.7359, 2.0416)
  line L180 (11.7359, 2.0416) -> (12.1373, 2.0416)
  line L181 (12.1373, 2.0416) -> (12.1373, -1.2749)
  spline S199 degree 2 poles (13.7608, -1.3289) (13.1896, -1.3289) (12.5618, -0.6883) (12.5618, -0.0965) knots 0 0 0 1 2 2 2
  spline S200 degree 2 poles (12.5618, -0.0965) (12.5618, 0.485) (13.1716, 1.1745) (13.663, 1.1745) knots 0 0 0 1 2 2 2
  spline S201 degree 2 poles (13.663, 1.1745) (13.8843, 1.1745) (14.2265, 1.0459) (14.3526, 0.9095) knots 0 0 0 1 2 2 2
  spline S202 degree 2 poles (14.3526, 0.9095) (14.4812, 0.7732) (14.6176, 0.3795) (14.6176, 0.0939) knots 0 0 0 1 2 2 2
  line L182 (14.6176, 0.0939) -> (14.6176, -0.1248)
  line L183 (14.6176, -0.1248) -> (12.9683, -0.1248)
  spline S203 degree 2 poles (12.9683, -0.1248) (12.9683, -0.539) (13.3851, -0.979) (13.7556, -0.979) knots 0 0 0 1 2 2 2
  spline S204 degree 2 poles (13.7556, -0.979) (13.8869, -0.979) (14.1416, -0.9198) (14.2445, -0.8735) knots 0 0 0 1 2 2 2
  spline S205 degree 2 poles (14.2445, -0.8735) (14.3526, -0.8221) (14.5018, -0.732) (14.5507, -0.6908) knots 0 0 0 1 2 2 2
  line L184 (14.5507, -0.6908) -> (14.5738, -0.6908)
  line L185 (14.5738, -0.6908) -> (14.5738, -1.1282)
  spline S206 degree 2 poles (14.5738, -1.1282) (14.5044, -1.1565) (14.2934, -1.2389) (14.2111, -1.262) knots 0 0 0 1 2 2 2
  spline S207 degree 2 poles (14.2111, -1.262) (14.0953, -1.2955) (13.9049, -1.3289) (13.7608, -1.3289) knots 0 0 0 1 2 2 2
  spline S208 degree 2 poles (14.2265, 0.1814) (14.2213, 0.3435) (14.1545, 0.5802) (14.0901, 0.66) knots 0 0 0 1 2 2 2
  spline S209 degree 2 poles (14.0901, 0.66) (14.0207, 0.75) (13.802, 0.8452) (13.6399, 0.8452) knots 0 0 0 1 2 2 2
  spline S210 degree 2 poles (13.6399, 0.8452) (13.4803, 0.8452) (13.2565, 0.75) (13.1639, 0.6574) knots 0 0 0 1 2 2 2
  spline S211 degree 2 poles (13.1639, 0.6574) (13.0738, 0.5622) (12.9812, 0.3332) (12.9683, 0.1814) knots 0 0 0 1 2 2 2
  line L186 (12.9683, 0.1814) -> (14.2265, 0.1814)
  line L187 (-9.9604, -6.5024) -> (-11.5093, -6.5024)
  line L188 (-11.5093, -6.5024) -> (-11.5093, -6.1783)
  line L189 (-11.5093, -6.1783) -> (-10.9329, -6.1783)
  line L190 (-10.9329, -6.1783) -> (-10.9329, -4.0504)
  line L191 (-10.9329, -4.0504) -> (-11.5093, -4.0504)
  line L192 (-11.5093, -4.0504) -> (-11.5093, -3.7597)
  spline S212 degree 2 poles (-11.5093, -3.7597) (-11.1825, -3.7597) (-10.8738, -3.5744) (-10.8532, -3.3172) knots 0 0 0 1 2 2 2
  line L193 (-10.8532, -3.3172) -> (-10.5238, -3.3172)
  line L194 (-10.5238, -3.3172) -> (-10.5238, -6.1783)
  line L195 (-10.5238, -6.1783) -> (-9.9604, -6.1783)
  line L196 (-9.9604, -6.1783) -> (-9.9604, -6.5024)
  spline S213 degree 2 poles (-7.4003, -4.9149) (-7.4003, -5.7692) (-7.8969, -6.5693) (-8.414, -6.5693) knots 0 0 0 1 2 2 2
  spline S214 degree 2 poles (-8.414, -6.5693) (-8.9389, -6.5693) (-9.4303, -5.7537) (-9.4303, -4.9175) knots 0 0 0 1 2 2 2
  spline S215 degree 2 poles (-9.4303, -4.9175) (-9.4303, -4.0582) (-8.9338, -3.2631) (-8.414, -3.2631) knots 0 0 0 1 2 2 2
  spline S216 degree 2 poles (-8.414, -3.2631) (-7.8917, -3.2631) (-7.4003, -4.0865) (-7.4003, -4.9149) knots 0 0 0 1 2 2 2
  spline S217 degree 2 poles (-7.9458, -5.8824) (-7.884, -5.7254) (-7.8326, -5.2417) (-7.8326, -4.9149) knots 0 0 0 1 2 2 2
  spline S218 degree 2 poles (-7.8326, -4.9149) (-7.8326, -4.5882) (-7.884, -4.107) (-7.9483, -3.9449) knots 0 0 0 1 2 2 2
  spline S219 degree 2 poles (-7.9483, -3.9449) (-8.0127, -3.7829) (-8.2365, -3.6156) (-8.414, -3.6156) knots 0 0 0 1 2 2 2
  spline S220 degree 2 poles (-8.414, -3.6156) (-8.5916, -3.6156) (-8.8206, -3.7829) (-8.8875, -3.9501) knots 0 0 0 1 2 2 2
  spline S221 degree 2 poles (-8.8875, -3.9501) (-8.9518, -4.1122) (-8.9981, -4.6062) (-8.9981, -4.9175) knots 0 0 0 1 2 2 2
  spline S222 degree 2 poles (-8.9981, -4.9175) (-8.9981, -5.252) (-8.9569, -5.6997) (-8.89, -5.8746) knots 0 0 0 1 2 2 2
  spline S223 degree 2 poles (-8.89, -5.8746) (-8.8283, -6.0393) (-8.5993, -6.2168) (-8.414, -6.2168) knots 0 0 0 1 2 2 2
  spline S224 degree 2 poles (-8.414, -6.2168) (-8.2391, -6.2168) (-8.0101, -6.0496) (-7.9458, -5.8824) knots 0 0 0 1 2 2 2
  line L197 (-5.6739, -3.1859) -> (-6.9166, -7.192)
  line L198 (-6.9166, -7.192) -> (-7.2768, -7.192)
  line L199 (-7.2768, -7.192) -> (-6.0392, -3.1859)
  line L200 (-6.0392, -3.1859) -> (-5.6739, -3.1859)
  line L201 (-3.3659, -6.5024) -> (-5.3239, -6.5024)
  line L202 (-5.3239, -6.5024) -> (-5.3239, -6.0522)
  spline S225 degree 2 poles (-5.3239, -6.0522) (-5.113, -5.8541) (-4.7373, -5.4861) (-4.5572, -5.288) knots 0 0 0 1 2 2 2
  spline S226 degree 2 poles (-4.5572, -5.288) (-4.1944, -4.8892) (-3.9294, -4.4106) (-3.9294, -4.1559) knots 0 0 0 1 2 2 2
  spline S227 degree 2 poles (-3.9294, -4.1559) (-3.9294, -4.0221) (-4.0117, -3.8214) (-4.0864, -3.7571) knots 0 0 0 1 2 2 2
  spline S228 degree 2 poles (-4.0864, -3.7571) (-4.161, -3.6928) (-4.3565, -3.6285) (-4.4749, -3.6285) knots 0 0 0 1 2 2 2
  spline S229 degree 2 poles (-4.4749, -3.6285) (-4.5881, -3.6285) (-4.8196, -3.6851) (-4.9251, -3.7288) knots 0 0 0 1 2 2 2
  spline S230 degree 2 poles (-4.9251, -3.7288) (-5.0152, -3.7648) (-5.1824, -3.8678) (-5.2339, -3.9038) knots 0 0 0 1 2 2 2
  line L203 (-5.2339, -3.9038) -> (-5.257, -3.9038)
  line L204 (-5.257, -3.9038) -> (-5.257, -3.4509)
  spline S231 degree 2 poles (-5.257, -3.4509) (-5.1258, -3.3866) (-4.655, -3.2605) (-4.444, -3.2605) knots 0 0 0 1 2 2 2
  spline S232 degree 2 poles (-4.444, -3.2605) (-3.9989, -3.2605) (-3.4972, -3.7314) (-3.4972, -4.1328) knots 0 0 0 1 2 2 2
  spline S233 degree 2 poles (-3.4972, -4.1328) (-3.4972, -4.3206) (-3.5846, -4.6345) (-3.6618, -4.7683) knots 0 0 0 1 2 2 2
  spline S234 degree 2 poles (-3.6618, -4.7683) (-3.739, -4.9072) (-3.9629, -5.18) (-4.0864, -5.3112) knots 0 0 0 1 2 2 2
  spline S235 degree 2 poles (-4.0864, -5.3112) (-4.287, -5.5299) (-4.7785, -5.9981) (-4.9251, -6.1345) knots 0 0 0 1 2 2 2
  line L205 (-4.9251, -6.1345) -> (-3.3659, -6.1345)
  line L206 (-3.3659, -6.1345) -> (-3.3659, -6.5024)
  spline S236 degree 2 poles (-2.0846, -3.6285) (-2.2004, -3.6285) (-2.4294, -3.6851) (-2.54, -3.7288) knots 0 0 0 1 2 2 2
  spline S237 degree 2 poles (-2.54, -3.7288) (-2.6429, -3.7726) (-2.7947, -3.8652) (-2.8539, -3.9064) knots 0 0 0 1 2 2 2
  line L207 (-2.8539, -3.9064) -> (-2.8797, -3.9064)
  line L208 (-2.8797, -3.9064) -> (-2.8797, -3.4561)
  spline S238 degree 2 poles (-2.8797, -3.4561) (-2.7407, -3.3815) (-2.2647, -3.2605) (-2.0512, -3.2605) knots 0 0 0 1 2 2 2
  spline S239 degree 2 poles (-2.0512, -3.2605) (-1.835, -3.2605) (-1.5134, -3.348) (-1.3822, -3.4407) knots 0 0 0 1 2 2 2
  spline S240 degree 2 poles (-1.3822, -3.4407) (-1.2433, -3.541) (-1.0992, -3.8317) (-1.0992, -4.0273) knots 0 0 0 1 2 2 2
  spline S241 degree 2 poles (-1.0992, -4.0273) (-1.0992, -4.2897) (-1.444, -4.686) (-1.6858, -4.7374) knots 0 0 0 1 2 2 2
  line L209 (-1.6858, -4.7374) -> (-1.6858, -4.7683)
  spline S242 degree 2 poles (-1.6858, -4.7683) (-1.5855, -4.7889) (-1.3565, -4.8815) (-1.2587, -4.9741) knots 0 0 0 1 2 2 2
  spline S243 degree 2 poles (-1.2587, -4.9741) (-1.1609, -5.0642) (-1.0374, -5.3523) (-1.0374, -5.5607) knots 0 0 0 1 2 2 2
  spline S244 degree 2 poles (-1.0374, -5.5607) (-1.0374, -5.7743) (-1.1841, -6.1371) (-1.3179, -6.276) knots 0 0 0 1 2 2 2
  spline S245 degree 2 poles (-1.3179, -6.276) (-1.4568, -6.4201) (-1.8505, -6.5693) (-2.1001, -6.5693) knots 0 0 0 1 2 2 2
  spline S246 degree 2 poles (-2.1001, -6.5693) (-2.3393, -6.5693) (-2.8076, -6.4536) (-2.9671, -6.3738) knots 0 0 0 1 2 2 2
  line L210 (-2.9671, -6.3738) -> (-2.9671, -5.9235)
  line L211 (-2.9671, -5.9235) -> (-2.9363, -5.9235)
  spline S247 degree 2 poles (-2.9363, -5.9235) (-2.8025, -6.0213) (-2.3496, -6.2014) (-2.1258, -6.2014) knots 0 0 0 1 2 2 2
  spline S248 degree 2 poles (-2.1258, -6.2014) (-1.9946, -6.2014) (-1.7321, -6.1191) (-1.6446, -6.0239) knots 0 0 0 1 2 2 2
  spline S249 degree 2 poles (-1.6446, -6.0239) (-1.5597, -5.9287) (-1.4697, -5.7023) (-1.4697, -5.5299) knots 0 0 0 1 2 2 2
  spline S250 degree 2 poles (-1.4697, -5.5299) (-1.4697, -5.3575) (-1.57, -5.1336) (-1.6601, -5.0693) knots 0 0 0 1 2 2 2
  spline S251 degree 2 poles (-1.6601, -5.0693) (-1.7501, -5.005) (-1.9946, -4.9561) (-2.1387, -4.9561) knots 0 0 0 1 2 2 2
  line L212 (-2.1387, -4.9561) -> (-2.3188, -4.9561)
  line L213 (-2.3188, -4.9561) -> (-2.3188, -4.6036)
  line L214 (-2.3188, -4.6036) -> (-2.1772, -4.6036)
  spline S252 degree 2 poles (-2.1772, -4.6036) (-1.8916, -4.6036) (-1.5314, -4.3309) (-1.5314, -4.071) knots 0 0 0 1 2 2 2
  spline S253 degree 2 poles (-1.5314, -4.071) (-1.5314, -3.9501) (-1.6241, -3.7777) (-1.6987, -3.7262) knots 0 0 0 1 2 2 2
  spline S254 degree 2 poles (-1.6987, -3.7262) (-1.7784, -3.6722) (-1.974, -3.6285) (-2.0846, -3.6285) knots 0 0 0 1 2 2 2
  line L215 (0.761, -3.1859) -> (-0.4817, -7.192)
  line L216 (-0.4817, -7.192) -> (-0.8419, -7.192)
  line L217 (-0.8419, -7.192) -> (0.3957, -3.1859)
  line L218 (0.3957, -3.1859) -> (0.761, -3.1859)
  line L219 (3.069, -6.5024) -> (1.111, -6.5024)
  line L220 (1.111, -6.5024) -> (1.111, -6.0522)
  spline S255 degree 2 poles (1.111, -6.0522) (1.3219, -5.8541) (1.6976, -5.4861) (1.8777, -5.288) knots 0 0 0 1 2 2 2
  spline S256 degree 2 poles (1.8777, -5.288) (2.2405, -4.8892) (2.5055, -4.4106) (2.5055, -4.1559) knots 0 0 0 1 2 2 2
  spline S257 degree 2 poles (2.5055, -4.1559) (2.5055, -4.0221) (2.4232, -3.8214) (2.3485, -3.7571) knots 0 0 0 1 2 2 2
  spline S258 degree 2 poles (2.3485, -3.7571) (2.2739, -3.6928) (2.0784, -3.6285) (1.96, -3.6285) knots 0 0 0 1 2 2 2
  spline S259 degree 2 poles (1.96, -3.6285) (1.8468, -3.6285) (1.6153, -3.6851) (1.5098, -3.7288) knots 0 0 0 1 2 2 2
  spline S260 degree 2 poles (1.5098, -3.7288) (1.4197, -3.7648) (1.2525, -3.8678) (1.201, -3.9038) knots 0 0 0 1 2 2 2
  line L221 (1.201, -3.9038) -> (1.1779, -3.9038)
  line L222 (1.1779, -3.9038) -> (1.1779, -3.4509)
  spline S261 degree 2 poles (1.1779, -3.4509) (1.3091, -3.3866) (1.7799, -3.2605) (1.9909, -3.2605) knots 0 0 0 1 2 2 2
  spline S262 degree 2 poles (1.9909, -3.2605) (2.436, -3.2605) (2.9377, -3.7314) (2.9377, -4.1328) knots 0 0 0 1 2 2 2
  spline S263 degree 2 poles (2.9377, -4.1328) (2.9377, -4.3206) (2.8503, -4.6345) (2.7731, -4.7683) knots 0 0 0 1 2 2 2
  spline S264 degree 2 poles (2.7731, -4.7683) (2.6959, -4.9072) (2.472, -5.18) (2.3485, -5.3112) knots 0 0 0 1 2 2 2
  spline S265 degree 2 poles (2.3485, -5.3112) (2.1479, -5.5299) (1.6564, -5.9981) (1.5098, -6.1345) knots 0 0 0 1 2 2 2
  line L223 (1.5098, -6.1345) -> (3.069, -6.1345)
  line L224 (3.069, -6.1345) -> (3.069, -6.5024)
  spline S266 degree 2 poles (5.4695, -4.9149) (5.4695, -5.7692) (4.9729, -6.5693) (4.4558, -6.5693) knots 0 0 0 1 2 2 2
  spline S267 degree 2 poles (4.4558, -6.5693) (3.9309, -6.5693) (3.4395, -5.7537) (3.4395, -4.9175) knots 0 0 0 1 2 2 2
  spline S268 degree 2 poles (3.4395, -4.9175) (3.4395, -4.0582) (3.936, -3.2631) (4.4558, -3.2631) knots 0 0 0 1 2 2 2
  spline S269 degree 2 poles (4.4558, -3.2631) (4.9781, -3.2631) (5.4695, -4.0865) (5.4695, -4.9149) knots 0 0 0 1 2 2 2
  spline S270 degree 2 poles (4.9241, -5.8824) (4.9858, -5.7254) (5.0373, -5.2417) (5.0373, -4.9149) knots 0 0 0 1 2 2 2
  spline S271 degree 2 poles (5.0373, -4.9149) (5.0373, -4.5882) (4.9858, -4.107) (4.9215, -3.9449) knots 0 0 0 1 2 2 2
  spline S272 degree 2 poles (4.9215, -3.9449) (4.8572, -3.7829) (4.6333, -3.6156) (4.4558, -3.6156) knots 0 0 0 1 2 2 2
  spline S273 degree 2 poles (4.4558, -3.6156) (4.2782, -3.6156) (4.0493, -3.7829) (3.9824, -3.9501) knots 0 0 0 1 2 2 2
  spline S274 degree 2 poles (3.9824, -3.9501) (3.918, -4.1122) (3.8717, -4.6062) (3.8717, -4.9175) knots 0 0 0 1 2 2 2
  spline S275 degree 2 poles (3.8717, -4.9175) (3.8717, -5.252) (3.9129, -5.6997) (3.9798, -5.8746) knots 0 0 0 1 2 2 2
  spline S276 degree 2 poles (3.9798, -5.8746) (4.0415, -6.0393) (4.2705, -6.2168) (4.4558, -6.2168) knots 0 0 0 1 2 2 2
  spline S277 degree 2 poles (4.4558, -6.2168) (4.6307, -6.2168) (4.8597, -6.0496) (4.9241, -5.8824) knots 0 0 0 1 2 2 2
  line L225 (7.834, -6.5024) -> (5.876, -6.5024)
  line L226 (5.876, -6.5024) -> (5.876, -6.0522)
  spline S278 degree 2 poles (5.876, -6.0522) (6.087, -5.8541) (6.4627, -5.4861) (6.6428, -5.288) knots 0 0 0 1 2 2 2
  spline S279 degree 2 poles (6.6428, -5.288) (7.0056, -4.8892) (7.2706, -4.4106) (7.2706, -4.1559) knots 0 0 0 1 2 2 2
  spline S280 degree 2 poles (7.2706, -4.1559) (7.2706, -4.0221) (7.1882, -3.8214) (7.1136, -3.7571) knots 0 0 0 1 2 2 2
  spline S281 degree 2 poles (7.1136, -3.7571) (7.039, -3.6928) (6.8435, -3.6285) (6.7251, -3.6285) knots 0 0 0 1 2 2 2
  spline S282 degree 2 poles (6.7251, -3.6285) (6.6119, -3.6285) (6.3803, -3.6851) (6.2748, -3.7288) knots 0 0 0 1 2 2 2
  spline S283 degree 2 poles (6.2748, -3.7288) (6.1848, -3.7648) (6.0175, -3.8678) (5.9661, -3.9038) knots 0 0 0 1 2 2 2
  line L227 (5.9661, -3.9038) -> (5.9429, -3.9038)
  line L228 (5.9429, -3.9038) -> (5.9429, -3.4509)
  spline S284 degree 2 poles (5.9429, -3.4509) (6.0742, -3.3866) (6.545, -3.2605) (6.756, -3.2605) knots 0 0 0 1 2 2 2
  spline S285 degree 2 poles (6.756, -3.2605) (7.2011, -3.2605) (7.7028, -3.7314) (7.7028, -4.1328) knots 0 0 0 1 2 2 2
  spline S286 degree 2 poles (7.7028, -4.1328) (7.7028, -4.3206) (7.6153, -4.6345) (7.5382, -4.7683) knots 0 0 0 1 2 2 2
  spline S287 degree 2 poles (7.5382, -4.7683) (7.461, -4.9072) (7.2371, -5.18) (7.1136, -5.3112) knots 0 0 0 1 2 2 2
  spline S288 degree 2 poles (7.1136, -5.3112) (6.9129, -5.5299) (6.4215, -5.9981) (6.2748, -6.1345) knots 0 0 0 1 2 2 2
  line L229 (6.2748, -6.1345) -> (7.834, -6.1345)
  line L230 (7.834, -6.1345) -> (7.834, -6.5024)
  spline S289 degree 2 poles (10.1831, -5.4939) (10.1831, -5.7228) (10.0365, -6.1139) (9.9027, -6.258) knots 0 0 0 1 2 2 2
  spline S290 degree 2 poles (9.9027, -6.258) (9.7689, -6.4021) (9.3701, -6.5693) (9.1231, -6.5693) knots 0 0 0 1 2 2 2
  spline S291 degree 2 poles (9.1231, -6.5693) (8.8967, -6.5693) (8.4541, -6.469) (8.292, -6.3892) knots 0 0 0 1 2 2 2
  line L231 (8.292, -6.3892) -> (8.292, -5.939)
  line L232 (8.292, -5.939) -> (8.3229, -5.939)
  spline S292 degree 2 poles (8.3229, -5.939) (8.3718, -5.975) (8.5545, -6.0676) (8.6651, -6.1088) knots 0 0 0 1 2 2 2
  spline S293 degree 2 poles (8.6651, -6.1088) (8.7912, -6.1525) (8.9996, -6.2014) (9.1308, -6.2014) knots 0 0 0 1 2 2 2
  spline S294 degree 2 poles (9.1308, -6.2014) (9.2594, -6.2014) (9.5013, -6.1088) (9.5888, -6.0084) knots 0 0 0 1 2 2 2
  spline S295 degree 2 poles (9.5888, -6.0084) (9.6685, -5.9132) (9.7509, -5.6611) (9.7509, -5.4913) knots 0 0 0 1 2 2 2
  spline S296 degree 2 poles (9.7509, -5.4913) (9.7509, -5.3215) (9.6582, -5.1053) (9.5708, -5.0333) knots 0 0 0 1 2 2 2
  spline S297 degree 2 poles (9.5708, -5.0333) (9.4807, -4.9535) (9.2131, -4.8866) (9.051, -4.8866) knots 0 0 0 1 2 2 2
  spline S298 degree 2 poles (9.051, -4.8866) (8.8761, -4.8866) (8.5287, -4.9407) (8.4232, -4.9638) knots 0 0 0 1 2 2 2
  line L233 (8.4232, -4.9638) -> (8.4232, -3.3274)
  line L234 (8.4232, -3.3274) -> (10.1651, -3.3274)
  line L235 (10.1651, -3.3274) -> (10.1651, -3.7005)
  line L236 (10.1651, -3.7005) -> (8.8323, -3.7005)
  line L237 (8.8323, -3.7005) -> (8.8323, -4.547)
  spline S299 degree 2 poles (8.8323, -4.547) (8.9095, -4.5367) (9.0588, -4.529) (9.1205, -4.529) knots 0 0 0 1 2 2 2
  spline S300 degree 2 poles (9.1205, -4.529) (9.3649, -4.529) (9.702, -4.6088) (9.8564, -4.7271) knots 0 0 0 1 2 2 2
  spline S301 degree 2 poles (9.8564, -4.7271) (10.0133, -4.8455) (10.1831, -5.2057) (10.1831, -5.4939) knots 0 0 0 1 2 2 2
  point P0 (0, 0)
  constraints: 2 other
emboss "Emboss1" sketch "Sketch2" operation cut depth 1.5 direction (0, 0, -1)
body "Solid1"
